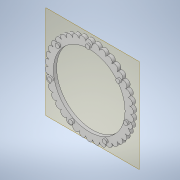
# Autodesk Inventor part: 20_Cube_Insert_CirAp_Wheel
Saved by Autodesk Inventor 2022 (Build 260153000, 153)
## iProperties
Created: 2019-10-23
Part Number: 20_Cube_Insert_CirAp_Wheel
Material: Generic
Document SubType Name: Modeling
Designer: marsikovabarbora
Density: 1 g/cm^3
Appearance: Default
Author: marsikovabarbora
Autodesk Inventor part; units mm, degrees
ref_plane "YZ Plane" through (0, 0, 0) normal (1, 0, 0) x (0, 1, 0)
ref_plane "XZ Plane" through (0, 0, 0) normal (0, 1, 0) x (-1, 0, 0)
ref_plane "XY Plane" through (0, 0, 0) normal (0, 0, 1) x (1, 0, 0)
ref_plane "Work Plane1" through (0, 0, -20) normal (0, 0, 1) x (1, 0, 0)
sketch "Sketch1" plane through (0, 0, -20) normal (0, 0, 1) x (1, 0, 0)
  circle A0 centre (0, 0) radius 20 construction
  line L0 (24.9006, -16.8) -> (24.9006, 16.8) construction
  line L1 (24.9006, 16.8) -> (21.2406, 16.8) construction
  line L2 (21.2406, 16.8) -> (16.8, 21.2406) construction
  line L3 (16.8, 21.2406) -> (16.8, 24.9006) construction
  line L4 (16.8, 24.9006) -> (-16.8, 24.9006) construction
  line L5 (-16.8, 24.9006) -> (-16.8, 21.2406) construction
  line L6 (-16.8, 21.2406) -> (-21.2406, 16.8) construction
  line L7 (-21.2406, 16.8) -> (-24.9006, 16.8) construction
  line L8 (-24.9006, 16.8) -> (-24.9006, -16.8) construction
  line L9 (-24.9006, -16.8) -> (-21.2406, -16.8) construction
  line L10 (-21.2406, -16.8) -> (-16.8, -21.2406) construction
  line L11 (-16.8, -21.2406) -> (-16.8, -24.9006) construction
  line L12 (-16.8, -24.9006) -> (16.8, -24.9006) construction
  line L13 (16.8, -24.9006) -> (16.8, -21.2406) construction
  line L14 (16.8, -21.2406) -> (21.2406, -16.8) construction
  line L15 (21.2406, -16.8) -> (24.9006, -16.8) construction
  line L16 (-36.4, 0) -> (36.4, 0) construction
  line L17 (0, -36.4) -> (0, 36.4) construction
  circle A1 centre (0, 0) radius 26
  circle A2 centre (0, 0) radius 21
  point P0 (0, 0)
  dimension "d0" = 52
  dimension "d1" = 42
  constraints: 2 centre point, 2 coincident
  measures "d0" diameter of A1
  measures "d1" diameter of A2
extrude "Extrusion1" add sketch "Sketch1" along normal blind 1.9
sketch "Sketch2" plane through (0, 0, -18.1) normal (0, 0, 1) x (1, 0, 0)
  circle A0 centre (0, 0) radius 21 construction
  circle A1 centre (0, 0) radius 26 construction
  line L0 (0, -36.4828) -> (0, 36.8971) construction
  arc A2 (2, 24) -> (0, 26) centre (0, 24) ccw
  line L1 (0, 24) -> (-2, 24) construction
  line L2 (0, 24) -> (2, 24) construction
  line L3 (0, 24) -> (2, 24) construction
  line L4 (-2, 24) -> (-2.1592, 25.9102)
  line L5 (2, 24) -> (2.1592, 25.9102)
  arc A3 (2.1592, 25.9102) -> (0, 26) centre (0, 0) ccw
  arc A4 (0, 26) -> (-2.1592, 25.9102) centre (0, 0) ccw
  arc A5 (0, 26) -> (-2, 24) centre (0, 24) ccw
  line L6 (0, 0) -> (-2.1592, 25.9102) construction
  line L7 (0, 0) -> (2.1592, 25.9102) construction
  point P0 (0, 0)
  dimension "d4" = 180
  dimension "d5" = 180
  dimension "d6" = 2
  constraints: 14 end point, 13 point on circle, 4 centre point, 3 collinear, 2 point on line, 1 coincident, 1 horizontal, 1 tangent
  measures "d4" angle of L1 L2
  measures "d5" angle of L1 L3
  measures "d6" radius of A2
extrude "Extrusion2" cut sketch "Sketch2" against normal up to next contours A5 L4 A4
mirror "Mirror1" about plane through (0, 0, 0) normal (1, 0, 0) of "Extrusion2"
pattern_circular "Circular Pattern1" count 38 over 360 about axis through (0, 0, -10) along (0, 0, 1) of "Extrusion2", "Mirror1"
sketch "Sketch3" plane through (0, 0, -18.1) normal (0, 0, 1) x (1, 0, 0)
  arc A0 (5.9445, 23.5204) -> (2.0147, 24.1761) centre (3.9503, 23.6727) ccw construction
  line L0 (2.0147, 24.1761) -> (2, 24) construction
  arc A1 (2, 24) -> (1.9973, 24.1039) centre (0, 24) ccw construction
  arc A2 (1.9973, 24.1039) -> (1.9775, 24.0019) centre (3.9503, 23.6727) ccw construction
  line L1 (1.9775, 24.0019) -> (1.9921, 24.178) construction
  arc A3 (1.9921, 24.178) -> (-1.9921, 24.178) centre (0, 24) ccw construction
  line L2 (-1.9921, 24.178) -> (-1.9775, 24.0019) construction
  arc A4 (-1.9775, 24.0019) -> (-1.9973, 24.1039) centre (-3.9503, 23.6727) ccw construction
  arc A5 (-1.9973, 24.1039) -> (-2, 24) centre (0, 24) ccw construction
  line L3 (-2, 24) -> (-2.0147, 24.1761) construction
  arc A6 (-2.0147, 24.1761) -> (-5.9445, 23.5204) centre (-3.9503, 23.6727) ccw construction
  line L4 (-5.9445, 23.5204) -> (-5.9012, 23.349) construction
  arc A7 (-5.9012, 23.349) -> (-5.9374, 23.4464) centre (-7.7928, 22.6996) ccw construction
  arc A8 (-5.9374, 23.4464) -> (-5.923, 23.3435) centre (-3.9503, 23.6727) ccw construction
  line L5 (-5.923, 23.3435) -> (-5.9665, 23.5148) construction
  arc A9 (-5.9665, 23.5148) -> (-9.7347, 22.2212) centre (-7.7928, 22.6996) ccw construction
  line L6 (-9.7347, 22.2212) -> (-9.6638, 22.0593) construction
  arc A10 (-9.6638, 22.0593) -> (-9.7156, 22.1493) centre (-11.4227, 21.1074) ccw construction
  arc A11 (-9.7156, 22.1493) -> (-9.6844, 22.0502) centre (-7.7928, 22.6996) ccw construction
  line L7 (-9.6844, 22.0502) -> (-9.7555, 22.212) construction
  arc A12 (-9.7555, 22.212) -> (-13.2594, 20.3158) centre (-11.4227, 21.1074) ccw construction
  line L8 (-13.2594, 20.3158) -> (-13.1628, 20.1678) construction
  arc A13 (-13.1628, 20.1678) -> (-13.2287, 20.2481) centre (-14.7411, 18.9394) ccw construction
  arc A14 (-13.2287, 20.2481) -> (-13.1817, 20.1555) centre (-11.4227, 21.1074) ccw construction
  line L9 (-13.1817, 20.1555) -> (-13.2784, 20.3034) construction
  arc A15 (-13.2784, 20.3034) -> (-16.4225, 17.8563) centre (-14.7411, 18.9394) ccw construction
  line L10 (-16.4225, 17.8563) -> (-16.3028, 17.7262) construction
  arc A16 (-16.3028, 17.7262) -> (-16.381, 17.7946) centre (-17.6574, 16.2548) ccw construction
  arc A17 (-16.381, 17.7946) -> (-16.3194, 17.7109) centre (-14.7411, 18.9394) ccw construction
  line L11 (-16.3194, 17.7109) -> (-16.4392, 17.8409) construction
  arc A18 (-16.4392, 17.8409) -> (-19.1375, 14.9097) centre (-17.6574, 16.2548) ccw construction
  line L12 (-19.1375, 14.9097) -> (-18.9981, 14.8011) construction
  arc A19 (-18.9981, 14.8011) -> (-19.0865, 14.8556) centre (-20.092, 13.1268) ccw construction
  arc A20 (-19.0865, 14.8556) -> (-19.0119, 14.7833) centre (-17.6574, 16.2548) ccw construction
  line L13 (-19.0119, 14.7833) -> (-19.1515, 14.8918) construction
  arc A21 (-19.1515, 14.8918) -> (-21.3306, 11.5564) centre (-20.092, 13.1268) ccw construction
  line L14 (-21.3306, 11.5564) -> (-21.1752, 11.4722) construction
  arc A22 (-21.1752, 11.4722) -> (-21.2714, 11.5115) centre (-21.9786, 9.6407) ccw construction
  arc A23 (-21.2714, 11.5115) -> (-21.1859, 11.4524) centre (-20.092, 13.1268) ccw construction
  line L15 (-21.1859, 11.4524) -> (-21.3414, 11.5365) construction
  arc A24 (-21.3414, 11.5365) -> (-22.9418, 7.8879) centre (-21.9786, 9.6407) ccw construction
  line L16 (-22.9418, 7.8879) -> (-22.7746, 7.8305) construction
  arc A25 (-22.7746, 7.8305) -> (-22.876, 7.8533) centre (-23.2656, 5.8917) ccw construction
  arc A26 (-22.876, 7.8533) -> (-22.782, 7.8091) centre (-21.9786, 9.6407) ccw construction
  line L17 (-22.782, 7.8091) -> (-22.9492, 7.8665) construction
  arc A27 (-22.9492, 7.8665) -> (-23.9272, 4.0042) centre (-23.2656, 5.8917) ccw construction
  line L18 (-23.9272, 4.0042) -> (-23.7529, 3.9751) construction
  arc A28 (-23.7529, 3.9751) -> (-23.8566, 3.981) centre (-23.918, 1.9819) ccw construction
  arc A29 (-23.8566, 3.981) -> (-23.7566, 3.9529) centre (-23.2656, 5.8917) ccw construction
  line L19 (-23.7566, 3.9529) -> (-23.9309, 3.9819) construction
  arc A30 (-23.9309, 3.9819) -> (-24.2599, 0.0113) centre (-23.918, 1.9819) ccw construction
  line L20 (-24.2599, 0.0113) -> (-24.0832, 0.0113) construction
  arc A31 (-24.0832, 0.0113) -> (-24.1865, 0) centre (-23.918, -1.9819) ccw construction
  arc A32 (-24.1865, 0) -> (-24.0832, -0.0113) centre (-23.918, 1.9819) ccw construction
  line L21 (-24.0832, -0.0113) -> (-24.2599, -0.0113) construction
  arc A33 (-24.2599, -0.0113) -> (-23.9309, -3.9819) centre (-23.918, -1.9819) ccw construction
  line L22 (-23.9309, -3.9819) -> (-23.7566, -3.9529) construction
  arc A34 (-23.7566, -3.9529) -> (-23.8566, -3.981) centre (-23.2656, -5.8917) ccw construction
  arc A35 (-23.8566, -3.981) -> (-23.7529, -3.9751) centre (-23.918, -1.9819) ccw construction
  line L23 (-23.7529, -3.9751) -> (-23.9272, -4.0042) construction
  arc A36 (-23.9272, -4.0042) -> (-22.9492, -7.8665) centre (-23.2656, -5.8917) ccw construction
  line L24 (-22.9492, -7.8665) -> (-22.782, -7.8091) construction
  arc A37 (-22.782, -7.8091) -> (-22.876, -7.8533) centre (-21.9786, -9.6407) ccw construction
  arc A38 (-22.876, -7.8533) -> (-22.7746, -7.8305) centre (-23.2656, -5.8917) ccw construction
  line L25 (-22.7746, -7.8305) -> (-22.9418, -7.8879) construction
  arc A39 (-22.9418, -7.8879) -> (-21.3414, -11.5365) centre (-21.9786, -9.6407) ccw construction
  line L26 (-21.3414, -11.5365) -> (-21.1859, -11.4524) construction
  arc A40 (-21.1859, -11.4524) -> (-21.2714, -11.5115) centre (-20.092, -13.1268) ccw construction
  arc A41 (-21.2714, -11.5115) -> (-21.1752, -11.4722) centre (-21.9786, -9.6407) ccw construction
  line L27 (-21.1752, -11.4722) -> (-21.3306, -11.5564) construction
  arc A42 (-21.3306, -11.5564) -> (-19.1515, -14.8918) centre (-20.092, -13.1268) ccw construction
  line L28 (-19.1515, -14.8918) -> (-19.0119, -14.7833) construction
  arc A43 (-19.0119, -14.7833) -> (-19.0865, -14.8556) centre (-17.6574, -16.2548) ccw construction
  arc A44 (-19.0865, -14.8556) -> (-18.9981, -14.8011) centre (-20.092, -13.1268) ccw construction
  line L29 (-18.9981, -14.8011) -> (-19.1375, -14.9097) construction
  arc A45 (-19.1375, -14.9097) -> (-16.4392, -17.8409) centre (-17.6574, -16.2548) ccw construction
  line L30 (-16.4392, -17.8409) -> (-16.3194, -17.7109) construction
  arc A46 (-16.3194, -17.7109) -> (-16.381, -17.7946) centre (-14.7411, -18.9394) ccw construction
  arc A47 (-16.381, -17.7946) -> (-16.3028, -17.7262) centre (-17.6574, -16.2548) ccw construction
  line L31 (-16.3028, -17.7262) -> (-16.4225, -17.8563) construction
  arc A48 (-16.4225, -17.8563) -> (-13.2784, -20.3034) centre (-14.7411, -18.9394) ccw construction
  line L32 (-13.2784, -20.3034) -> (-13.1817, -20.1555) construction
  arc A49 (-13.1817, -20.1555) -> (-13.2287, -20.2481) centre (-11.4227, -21.1074) ccw construction
  arc A50 (-13.2287, -20.2481) -> (-13.1628, -20.1678) centre (-14.7411, -18.9394) ccw construction
  line L33 (-13.1628, -20.1678) -> (-13.2594, -20.3158) construction
  arc A51 (-13.2594, -20.3158) -> (-9.7555, -22.212) centre (-11.4227, -21.1074) ccw construction
  line L34 (-9.7555, -22.212) -> (-9.6844, -22.0502) construction
  arc A52 (-9.6844, -22.0502) -> (-9.7156, -22.1493) centre (-7.7928, -22.6996) ccw construction
  arc A53 (-9.7156, -22.1493) -> (-9.6638, -22.0593) centre (-11.4227, -21.1074) ccw construction
  line L35 (-9.6638, -22.0593) -> (-9.7347, -22.2212) construction
  arc A54 (-9.7347, -22.2212) -> (-5.9665, -23.5148) centre (-7.7928, -22.6996) ccw construction
  line L36 (-5.9665, -23.5148) -> (-5.923, -23.3435) construction
  arc A55 (-5.923, -23.3435) -> (-5.9374, -23.4464) centre (-3.9503, -23.6727) ccw construction
  arc A56 (-5.9374, -23.4464) -> (-5.9012, -23.349) centre (-7.7928, -22.6996) ccw construction
  line L37 (-5.9012, -23.349) -> (-5.9445, -23.5204) construction
  arc A57 (-5.9445, -23.5204) -> (-2.0147, -24.1761) centre (-3.9503, -23.6727) ccw construction
  line L38 (-2.0147, -24.1761) -> (-2, -24) construction
  arc A58 (-2, -24) -> (-1.9973, -24.1039) centre (0, -24) ccw construction
  arc A59 (-1.9973, -24.1039) -> (-1.9775, -24.0019) centre (-3.9503, -23.6727) ccw construction
  line L39 (-1.9775, -24.0019) -> (-1.9921, -24.178) construction
  arc A60 (-1.9921, -24.178) -> (1.9921, -24.178) centre (0, -24) ccw construction
  line L40 (1.9921, -24.178) -> (1.9775, -24.0019) construction
  arc A61 (1.9775, -24.0019) -> (1.9973, -24.1039) centre (3.9503, -23.6727) ccw construction
  arc A62 (1.9973, -24.1039) -> (2, -24) centre (0, -24) ccw construction
  line L41 (2, -24) -> (2.0147, -24.1761) construction
  arc A63 (2.0147, -24.1761) -> (5.9445, -23.5204) centre (3.9503, -23.6727) ccw construction
  line L42 (5.9445, -23.5204) -> (5.9012, -23.349) construction
  arc A64 (5.9012, -23.349) -> (5.9374, -23.4464) centre (7.7928, -22.6996) ccw construction
  arc A65 (5.9374, -23.4464) -> (5.923, -23.3435) centre (3.9503, -23.6727) ccw construction
  line L43 (5.923, -23.3435) -> (5.9665, -23.5148) construction
  arc A66 (5.9665, -23.5148) -> (9.7347, -22.2212) centre (7.7928, -22.6996) ccw construction
  line L44 (9.7347, -22.2212) -> (9.6638, -22.0593) construction
  arc A67 (9.6638, -22.0593) -> (9.7156, -22.1493) centre (11.4227, -21.1074) ccw construction
  arc A68 (9.7156, -22.1493) -> (9.6844, -22.0502) centre (7.7928, -22.6996) ccw construction
  line L45 (9.6844, -22.0502) -> (9.7555, -22.212) construction
  arc A69 (9.7555, -22.212) -> (13.2594, -20.3158) centre (11.4227, -21.1074) ccw construction
  line L46 (13.2594, -20.3158) -> (13.1628, -20.1678) construction
  arc A70 (13.1628, -20.1678) -> (13.2287, -20.2481) centre (14.7411, -18.9394) ccw construction
  arc A71 (13.2287, -20.2481) -> (13.1817, -20.1555) centre (11.4227, -21.1074) ccw construction
  line L47 (13.1817, -20.1555) -> (13.2784, -20.3034) construction
  arc A72 (13.2784, -20.3034) -> (16.4225, -17.8563) centre (14.7411, -18.9394) ccw construction
  line L48 (16.4225, -17.8563) -> (16.3028, -17.7262) construction
  arc A73 (16.3028, -17.7262) -> (16.381, -17.7946) centre (17.6574, -16.2548) ccw construction
  arc A74 (16.381, -17.7946) -> (16.3194, -17.7109) centre (14.7411, -18.9394) ccw construction
  line L49 (16.3194, -17.7109) -> (16.4392, -17.8409) construction
  arc A75 (16.4392, -17.8409) -> (19.1375, -14.9097) centre (17.6574, -16.2548) ccw construction
  line L50 (19.1375, -14.9097) -> (18.9981, -14.8011) construction
  arc A76 (18.9981, -14.8011) -> (19.0865, -14.8556) centre (20.092, -13.1268) ccw construction
  arc A77 (19.0865, -14.8556) -> (19.0119, -14.7833) centre (17.6574, -16.2548) ccw construction
  line L51 (19.0119, -14.7833) -> (19.1515, -14.8918) construction
  arc A78 (19.1515, -14.8918) -> (21.3306, -11.5564) centre (20.092, -13.1268) ccw construction
  line L52 (21.3306, -11.5564) -> (21.1752, -11.4722) construction
  arc A79 (21.1752, -11.4722) -> (21.2714, -11.5115) centre (21.9786, -9.6407) ccw construction
  arc A80 (21.2714, -11.5115) -> (21.1859, -11.4524) centre (20.092, -13.1268) ccw construction
  line L53 (21.1859, -11.4524) -> (21.3414, -11.5365) construction
  arc A81 (21.3414, -11.5365) -> (22.9418, -7.8879) centre (21.9786, -9.6407) ccw construction
  line L54 (22.9418, -7.8879) -> (22.7746, -7.8305) construction
  arc A82 (22.7746, -7.8305) -> (22.876, -7.8533) centre (23.2656, -5.8917) ccw construction
  arc A83 (22.876, -7.8533) -> (22.782, -7.8091) centre (21.9786, -9.6407) ccw construction
  line L55 (22.782, -7.8091) -> (22.9492, -7.8665) construction
  arc A84 (22.9492, -7.8665) -> (23.9272, -4.0042) centre (23.2656, -5.8917) ccw construction
  line L56 (23.9272, -4.0042) -> (23.7529, -3.9751) construction
  arc A85 (23.7529, -3.9751) -> (23.8566, -3.981) centre (23.918, -1.9819) ccw construction
  arc A86 (23.8566, -3.981) -> (23.7566, -3.9529) centre (23.2656, -5.8917) ccw construction
  line L57 (23.7566, -3.9529) -> (23.9309, -3.9819) construction
  arc A87 (23.9309, -3.9819) -> (24.2599, -0.0113) centre (23.918, -1.9819) ccw construction
  line L58 (24.2599, -0.0113) -> (24.0832, -0.0113) construction
  arc A88 (24.0832, -0.0113) -> (24.1865, 0) centre (23.918, 1.9819) ccw construction
  arc A89 (24.1865, 0) -> (24.0832, 0.0113) centre (23.918, -1.9819) ccw construction
  line L59 (24.0832, 0.0113) -> (24.2599, 0.0113) construction
  arc A90 (24.2599, 0.0113) -> (23.9309, 3.9819) centre (23.918, 1.9819) ccw construction
  line L60 (23.9309, 3.9819) -> (23.7566, 3.9529) construction
  arc A91 (23.7566, 3.9529) -> (23.8566, 3.981) centre (23.2656, 5.8917) ccw construction
  arc A92 (23.8566, 3.981) -> (23.7529, 3.9751) centre (23.918, 1.9819) ccw construction
  line L61 (23.7529, 3.9751) -> (23.9272, 4.0042) construction
  arc A93 (23.9272, 4.0042) -> (22.9492, 7.8665) centre (23.2656, 5.8917) ccw construction
  line L62 (22.9492, 7.8665) -> (22.782, 7.8091) construction
  arc A94 (22.782, 7.8091) -> (22.876, 7.8533) centre (21.9786, 9.6407) ccw construction
  arc A95 (22.876, 7.8533) -> (22.7746, 7.8305) centre (23.2656, 5.8917) ccw construction
  line L63 (22.7746, 7.8305) -> (22.9418, 7.8879) construction
  arc A96 (22.9418, 7.8879) -> (21.3414, 11.5365) centre (21.9786, 9.6407) ccw construction
  line L64 (21.3414, 11.5365) -> (21.1859, 11.4524) construction
  arc A97 (21.1859, 11.4524) -> (21.2714, 11.5115) centre (20.092, 13.1268) ccw construction
  arc A98 (21.2714, 11.5115) -> (21.1752, 11.4722) centre (21.9786, 9.6407) ccw construction
  line L65 (21.1752, 11.4722) -> (21.3306, 11.5564) construction
  arc A99 (21.3306, 11.5564) -> (19.1515, 14.8918) centre (20.092, 13.1268) ccw construction
  line L66 (19.1515, 14.8918) -> (19.0119, 14.7833) construction
  arc A100 (19.0119, 14.7833) -> (19.0865, 14.8556) centre (17.6574, 16.2548) ccw construction
  arc A101 (19.0865, 14.8556) -> (18.9981, 14.8011) centre (20.092, 13.1268) ccw construction
  line L67 (18.9981, 14.8011) -> (19.1375, 14.9097) construction
  arc A102 (19.1375, 14.9097) -> (16.4392, 17.8409) centre (17.6574, 16.2548) ccw construction
  line L68 (16.4392, 17.8409) -> (16.3194, 17.7109) construction
  arc A103 (16.3194, 17.7109) -> (16.381, 17.7946) centre (14.7411, 18.9394) ccw construction
  arc A104 (16.381, 17.7946) -> (16.3028, 17.7262) centre (17.6574, 16.2548) ccw construction
  line L69 (16.3028, 17.7262) -> (16.4225, 17.8563) construction
  arc A105 (16.4225, 17.8563) -> (13.2784, 20.3034) centre (14.7411, 18.9394) ccw construction
  line L70 (13.2784, 20.3034) -> (13.1817, 20.1555) construction
  arc A106 (13.1817, 20.1555) -> (13.2287, 20.2481) centre (11.4227, 21.1074) ccw construction
  arc A107 (13.2287, 20.2481) -> (13.1628, 20.1678) centre (14.7411, 18.9394) ccw construction
  line L71 (13.1628, 20.1678) -> (13.2594, 20.3158) construction
  arc A108 (13.2594, 20.3158) -> (9.7555, 22.212) centre (11.4227, 21.1074) ccw construction
  line L72 (9.7555, 22.212) -> (9.6844, 22.0502) construction
  arc A109 (9.6844, 22.0502) -> (9.7156, 22.1493) centre (7.7928, 22.6996) ccw construction
  arc A110 (9.7156, 22.1493) -> (9.6638, 22.0593) centre (11.4227, 21.1074) ccw construction
  line L73 (9.6638, 22.0593) -> (9.7347, 22.2212) construction
  arc A111 (9.7347, 22.2212) -> (5.9665, 23.5148) centre (7.7928, 22.6996) ccw construction
  line L74 (5.9665, 23.5148) -> (5.923, 23.3435) construction
  arc A112 (5.923, 23.3435) -> (5.9374, 23.4464) centre (3.9503, 23.6727) ccw construction
  arc A113 (5.9374, 23.4464) -> (5.9012, 23.349) centre (7.7928, 22.6996) ccw construction
  line L75 (5.9012, 23.349) -> (5.9445, 23.5204) construction
  circle A114 centre (0, 0) radius 21 construction
  line L76 (-36.506, 0) -> (36.506, 0) construction
  line L77 (0, -36.4) -> (0, 36.4) construction
  circle A115 centre (0, 22.75) radius 1.25
  point P0 (0, 0)
  dimension "d12" = 2.5
  constraints: 1 point on line, 1 vertical alignment, 2 other
extrude "Extrusion3" add sketch "Sketch3" along normal blind 1
pattern_circular "Circular Pattern2" count 7 over 360 about axis through (0, 0, -10) along (0, 0, 1) of "Extrusion3"
body "Solid1"
